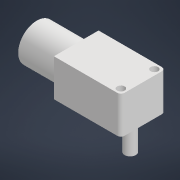
# Autodesk Inventor part: MotorRightAngle
Saved by Autodesk Inventor 2022 (Build 260153000, 153)
## iProperties
Created: 2022-04-02
Part Number: MotorRightAngle
Material: Generic
Document SubType Name: Modeling
Designer: Vinicius Miguel
Density: 1 g/cm^3
Appearance: Default
Author: Vinicius Miguel
Autodesk Inventor part; units mm, degrees
ref_plane "YZ Plane" through (0, 0, 0) normal (1, 0, 0) x (0, 1, 0)
ref_plane "XZ Plane" through (0, 0, 0) normal (0, 1, 0) x (-1, 0, 0)
ref_plane "XY Plane" through (0, 0, 0) normal (0, 0, 1) x (1, 0, 0)
sketch "Sketch1" plane through (0, 0, 0) normal (0, 1, 0) x (-1, 0, 0)
  circle A0 centre (0, 0) radius 1.5
  dimension "d0" = 3
  constraints: 1 centre point, 1 coincident
  measures "d0" diameter of A0
extrude "Extrusion1" add sketch "Sketch1" against normal blind 8
sketch "Sketch2" plane through (0, 0, 0) normal (0, 1, 0) x (1, 0, 0)
  line L0 (-14.5, -6) -> (3.5, -6)
  line L1 (3.5, -6) -> (3.5, 6)
  line L2 (3.5, 6) -> (-14.5, 6)
  line L3 (-14.5, 6) -> (-14.5, -6)
  line L4 (-14.5, -6) -> (3.5, 6) construction
  line L5 (3.5, -6) -> (-14.5, 6) construction
  point P0 (0, 0)
  point P1 (-5.5, 0)
  point P2 (-5.5, 0)
  dimension "d3" = 18
  dimension "d4" = 12
  dimension "d5" = 3.5
  constraints: 12 end point, 3 midpoint, 2 parallel, 1 horizontal, 1 horizontal alignment, 1 perpendicular
  measures "d3" distance of L1.end L2.end
  measures "d4" distance of L0.end L1.end
  measures "d5" distance from line of L1 point (0, 0)
extrude "Extrusion2" add sketch "Sketch2" along normal blind 10
sketch "Sketch3" plane through (-14.5, 0, -6) normal (-1, 0, 0) x (0, 0, 1)
  line L0 (0, 0) -> (12, 0) projected
  line L1 (12, 0) -> (12, 10) projected
  line L2 (0, 10) -> (12, 10) projected
  line L3 (0, 0) -> (0, 10) projected
  circle A0 centre (6, 5) radius 5
  point P0 (6, 0)
  point P1 (0, 5)
  point P2 (6, 10)
  dimension "d8" = 10
  constraints: 2 midpoint, 1 centre point, 1 horizontal alignment, 1 vertical alignment
  measures "d8" diameter of A0
extrude "Extrusion3" add sketch "Sketch3" along normal blind 10.6 contours A0
fillet "Fillet1" radius 1 2 edges at (3.5, 5, -6) (3.5, 5, 6)
sketch "Sketch4" plane through (0, 10, 0) normal (0, 1, 0) x (1, 0, 0)
  line L0 (2.5, 6) -> (-14.5, 6) projected
  line L1 (-14.5, -6) -> (2.5, -6) projected
  line L2 (3.5, -5) -> (3.5, 5) projected
  point P0 (0, 0)
  point P1 (2, 4.5)
  point P2 (2, -4.5)
  dimension "d12" = 1.5
  dimension "d13" = 1.5
  dimension "d14" = 1.5
  constraints: 1 vertical alignment
  measures "d12" distance from line of point (2, 4.5) L0
  measures "d13" distance from line of L1 point (2, -4.5)
  measures "d14" distance from line of L2 point (2, 4.5)
hole "Hole1" at (2, 10, -4.5) at (2, 10, 4.5) direction (0, -1, 0) diameter 2 end through all
equation "\"d13\" = d12"
equation "\"d14\" = d12"
body "Solid1"
